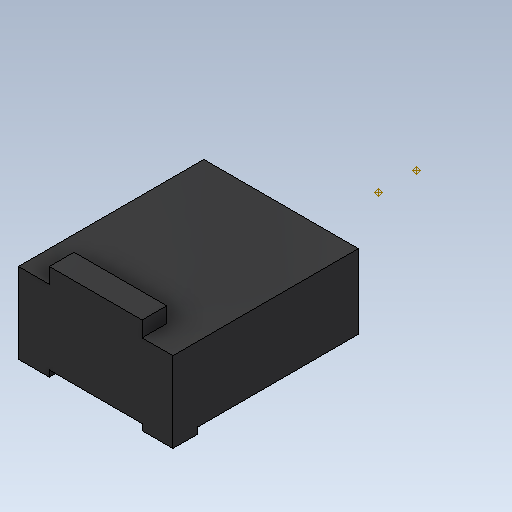
# Autodesk Inventor part: 10 Pin DR
Saved by Autodesk Inventor 2020.1 (Build 241239000, 239)
## iProperties
GlobalPropertyList: <PropertyList/>
Created: 2005-10-04
Part Number: 10 Pin DR
Document SubType Name: Modeling
Designer: Autodesk
Density: 1 g/cm^3
Mass: 1.20478 g
Surface Area: 7.61547 cm^2
Volume: 1.20478 cm^3
Categories: <MemberInstance><Categories><Category DisplayName="" Mnemonic="CABLEANDHARNESS" InternalName="e4a7e005-5e42-4d16-b293-125e7f0d0512"><Category DisplayName="" Mnemonic="CONNECTORS" InternalName="6f634eba-a678-4820-a31d-2c2d5ee6728e"><CategoryParameter DisplayName="" Mnemonic="REFDES" InternalName="c3740e8c-60ab-4d5d-8584-52b73222f2f0"/><Category DisplayName="" Mnemonic="DISCRETEWIRE" InternalName="9a3407de-09b2-4cdb-8c40-9708d5144a28"/></Category></Category></Categories><FamilyTemplate><FamilyTemplateParameters></FamilyTemplateParameters></FamilyTemplate><CategoryParameterMap><ParamToTemplateMap><ParamToTemplate CategoryParameter="//CategoryParameter[@InternalName='c3740e8c-60ab-4d5d-8584-52b73222f2f0']" ConstantValue=""/></ParamToTemplateMap></CategoryParameterMap></MemberInstance>
Material: Generic
Appearance: Dark Gray
Total Footprint: 0.000 kg
Author: Autodesk
Autodesk Inventor part; units mm, degrees
ref_plane "YZ Plane" through (0, 0, 0) normal (1, 0, 0) x (0, 1, 0)
ref_plane "XZ Plane" through (0, 0, 0) normal (0, 1, 0) x (-1, 0, 0)
ref_plane "XY Plane" through (0, 0, 0) normal (0, 0, 1) x (1, 0, 0)
sketch "Sketch1" plane through (0, 0, 0) normal (0, 0, 1) x (1, 0, 0)
  line L0 (-6.35, 3.048) -> (6.35, 3.048)
  line L1 (6.35, 3.048) -> (6.35, -3.048)
  line L2 (6.35, -3.048) -> (-6.35, -3.048)
  line L3 (-6.35, -3.048) -> (-6.35, 3.048)
  point P0 (0, 0)
  point P1 (0, -3.048)
  point P2 (-6.35, 0)
  dimension "d0" = 12.7
  dimension "d1" = 6.096
  constraints: 8 end point, 2 midpoint, 2 parallel, 1 horizontal, 1 horizontal alignment, 1 perpendicular, 1 vertical alignment
  measures "d0" distance of L1.end L2.end
  measures "d1" distance of L2.end L0.start
extrude "Extrusion1" add sketch "Sketch1" along normal blind 15.24
sketch "Sketch2" plane through (-6.35, 3.048, 0) normal (0, 1, 0) x (1, 0, 0)
  line L0 (0, -15.24) -> (12.7, -15.24) projected
  line L1 (2.54, -13.208) -> (10.16, -13.208)
  line L2 (10.16, -13.208) -> (10.16, -15.24)
  line L3 (10.16, -15.24) -> (2.54, -15.24)
  line L4 (2.54, -15.24) -> (2.54, -13.208)
  point P0 (6.35, -15.24)
  dimension "d4" = 7.62
  dimension "d5" = 2.032
  constraints: 8 end point, 2 midpoint, 2 parallel, 1 horizontal, 1 perpendicular
  measures "d4" distance of L1.start L1.end
  measures "d5" distance of L3.end L1.start
extrude "Extrusion2" add sketch "Sketch2" along normal blind 1.27
sketch "Sketch3" plane through (-6.35, -3.048, 0) normal (0, -1, 0) x (1, 0, 0)
  line L0 (0, 15.24) -> (2.54, 15.24)
  line L1 (2.54, 15.24) -> (2.54, 13.208)
  line L2 (2.54, 13.208) -> (0, 13.208)
  line L3 (0, 13.208) -> (0, 15.24)
  line L4 (12.7, 15.24) -> (10.16, 15.24)
  line L5 (10.16, 15.24) -> (10.16, 13.208)
  line L6 (10.16, 13.208) -> (12.7, 13.208)
  line L7 (12.7, 13.208) -> (12.7, 15.24)
  dimension "d8" = 2.54
  dimension "d9" = 2.54
  dimension "d10" = 2.032
  dimension "d11" = 2.032
  constraints: 16 end point, 4 parallel, 2 horizontal, 2 perpendicular
  measures "d8" distance of L1.end L2.end
  measures "d9" distance of L5.end L6.end
  measures "d10" distance of L0.end L1.end
  measures "d11" distance of L4.end L5.end
extrude "Extrusion3" add sketch "Sketch3" along normal blind 0.508
sketch "Sketch4" plane through (0, 0, 0) normal (0, 0, -1) x (-1, 0, 0)
  line L0 (6.35, 3.048) -> (-6.35, 3.048) projected
  line L1 (-6.35, 3.048) -> (-6.35, -3.048) projected
  line L2 (-6.35, -3.048) -> (6.35, -3.048) projected
  line L3 (6.35, -3.048) -> (6.35, 3.048) projected
  point P0 (-5.08, 1.27)
  point P1 (-2.54, 1.27)
  point P2 (2.54, 1.27)
  point P3 (5.08, 1.27)
  point P4 (-5.08, -1.27)
  point P5 (-2.54, -1.27)
  point P6 (2.54, -1.27)
  point P7 (5.08, -1.27)
  point P8 (0, 3.048)
  point P9 (0, 1.27)
  point P10 (0, -1.27)
  point P11 (0, 1.27)
  point P12 (0, -1.27)
  dimension "d14" = 1.27
  dimension "d15" = 1.778
  dimension "d16" = 1.27
  dimension "d17" = 1.778
  dimension "d18" = 2.54
  dimension "d19" = 2.54
  dimension "d20" = 2.54
  dimension "d21" = 2.54
  constraints: 10 horizontal alignment, 6 vertical alignment, 1 midpoint
  measures "d14" distance from line of L1 point (-5.08, 1.27)
  measures "d15" distance from line of L0 point (-5.08, 1.27)
  measures "d16" distance from line of point (5.08, -1.27) L3
  measures "d17" distance from line of L2 point (5.08, -1.27)
  measures "d18" distance of point (-5.08, 1.27) point (-2.54, 1.27)
  measures "d19" distance of point (5.08, 1.27) point (2.54, 1.27)
  measures "d20" distance of point (2.54, 1.27) point (0, 1.27)
  measures "d21" distance of point (-2.54, 1.27) point (0, 1.27)
body "Solid1"
